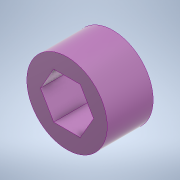
# Autodesk Inventor part: Churro Spacer
Saved by Autodesk Inventor 2020 (Build 240168000, 168)
## iProperties
Created: 2022-09-23
Part Number: Churro Spacer
Material: Generic
Document SubType Name: Modeling
Designer: Jason
Density: 1 g/cm^3
Appearance: Smooth - Purple
Author: Jason
Autodesk Inventor part; units mm, degrees
ref_plane "YZ Plane" through (0, 0, 0) normal (1, 0, 0) x (0, 1, 0)
ref_plane "XZ Plane" through (0, 0, 0) normal (0, 1, 0) x (-1, 0, 0)
ref_plane "XY Plane" through (0, 0, 0) normal (0, 0, 1) x (1, 0, 0)
sketch "Sketch1" plane through (0, 0, 0) normal (0, 0, 1) x (1, 0, 0)
  circle A0 centre (0, 0) radius 11.1125
  line L0 (0, 0) -> (7.3323, 0)
  line L1 (-3.7029, 6.35) -> (3.6662, 6.35)
  line L2 (3.6662, 6.35) -> (7.3323, 0)
  line L3 (7.3323, 0) -> (3.6662, -6.35)
  line L4 (3.6662, -6.35) -> (-3.6662, -6.35)
  line L5 (-3.6662, -6.35) -> (-7.3138, -0.0322)
  line L6 (-7.3138, -0.0322) -> (-3.7029, 6.35)
  line L7 (0, 0) -> (0, 6.35)
  line L8 (0, 0) -> (0, -6.35)
  line L9 (0, 0) -> (-5.4993, 3.175)
  line L10 (0, 0) -> (5.4993, -3.175)
  line L11 (0, 0) -> (5.4993, 3.175)
  line L12 (0, 0) -> (-5.4993, -3.175)
  dimension "d0" = 22.225
  dimension "d16" = 12.7
  dimension "d17" = 12.7
  dimension "d18" = 0.5
  dimension "d19" = 6.35
  dimension "d20" = 6.35
  dimension "d21" = 6.35
  dimension "d22" = 6.35
  dimension "d23" = 60
  dimension "d24" = 60
  dimension "d25" = 6.35
  dimension "d26" = 6.35
  dimension "d27" = 60
  dimension "d28" = 60
  constraints: 26 end point, 3 midpoint, 2 point on line, 2 vertical, 1 centre point, 1 coincident, 1 horizontal, 1 parallel, 1 perpendicular
  measures "d0" diameter of A0
  measures "d16" distance between parallel lines of L5 L2
  measures "d17" distance between parallel lines of L4 L1
  measures "d18" angle of L3 L6
  measures "d19" distance of L0.start L7.end
  measures "d20" distance of L0.start L8.end
  measures "d21" distance of L0.start L9.end
  measures "d22" distance of L0.start L10.end
  measures "d23" angle of L7 L9
  measures "d24" angle of L8 L10
  measures "d25" distance of L0.start L11.end
  measures "d26" distance of L0.start L12.end
  measures "d27" angle of L8 L12
  measures "d28" angle of L7 L11
extrude "Extrusion1" add sketch "Sketch1" along normal blind 12.7
body "Solid1"
